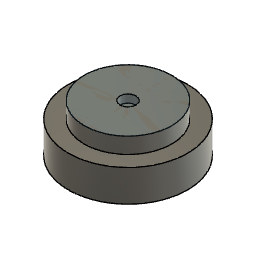
Base do meio v3 (Autodesk Fusion 360 design; units mm, degrees)
Autodesk Fusion 360 part; units mm, degrees
sketch "Sketch1" plane through (0, 0, 0) normal (0, 1, 0) x (1, 0, 0)
  circle A0 centre (0, 0) radius 75
  dimension "d1" = 150
  constraint coincident A0.centre origin
  measures "d1" diameter of A0
extrude "Extrude1" add sketch "Sketch1" along normal blind 40 makes body 1
sketch "Sketch2" plane through (0, 40, 0) normal (0, 1, 0) x (-1, 0, 0)
  circle A0 centre (0, 0) radius 75
  circle A1 centre (0, 0) radius 55
  dimension "d4" = 110
  constraint coincident A0.centre A1.centre
  measures "d4" diameter of A1
extrude "Extrude2" add sketch "Sketch2" along normal blind 20 contours A1 bodies 1
sketch "Sketch3" plane through (0, 60, 0) normal (0, 1, 0) x (-1, 0, 0)
  circle A0 centre (0, 0) radius 55
sketch "Sketch4" plane through (0, 60, 0) normal (0, 1, 0) x (-1, 0, 0)
  circle A0 centre (0, 0) radius 10
  dimension "d7" = 20
  constraint coincident A0.centre origin
  measures "d7" diameter of A0
extrude "Extrude3" cut sketch "Sketch4" against normal blind 10 bodies 1
sketch "Sketch6" plane through (0, 0, 0) normal (0, -1, 0) x (1, 0, 0)
  circle A0 centre (0, 0) radius 75
  circle A1 centre (0, 0) radius 12.5
  dimension "d10" = 25
  constraint concentric A0 A1
  measures "d10" diameter of A1
extrude "Extrude4" cut sketch "Sketch6" against normal blind 30 contours A1 bodies 1
copy_body "Body->Comp1" bodies 1 removing the originals makes body 2 in component "Component"
component "Component" placed x (1, 0, 0) y (0, 1, 0) z (0, 0, 1) at (0, 0, 0)
